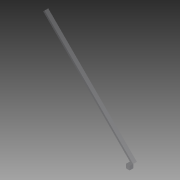
# Autodesk Inventor part: Mount
Saved by Autodesk Inventor 2013 (Build 170138000, 138)
## iProperties
Created: 2013-01-28
Part Number: Mount
Material: Polycarbonate, Clear
Document SubType Name: Modeling
Designer: Andrew Toennies
Density: 1.2 g/cm^3
Mass: 4.54796 g
Surface Area: 35.2548 cm^2
Volume: 3.78996 cm^3
Author: Andrew Toennies
Autodesk Inventor part; units mm, degrees
ref_plane "YZ Plane" through (0, 0, 0) normal (1, 0, 0) x (0, 1, 0)
ref_plane "XZ Plane" through (0, 0, 0) normal (0, 1, 0) x (-1, 0, 0)
ref_plane "XY Plane" through (0, 0, 0) normal (0, 0, 1) x (1, 0, 0)
sketch "Sketch1" plane through (0, 0, 0) normal (0, 0, 1) x (1, 0, 0)
  line L0 (-136.6846, 154.6451) -> (-138.9296, 152.4)
  line L1 (0, 0) -> (0, -6.35)
  line L2 (0, -6.35) -> (6.35, -6.35)
  line L3 (6.35, -6.35) -> (6.35, 0)
  line L4 (6.35, 0) -> (10.6475, 4.2975)
  line L5 (-108.1483, 123.0933) -> (17.5753, -2.6303) projected
  line L6 (10.6475, 4.2975) -> (-108.1483, 123.0933)
  line L7 (-108.1483, 123.0933) -> (-110.3933, 120.8483)
  line L8 (-110.3933, 120.8483) -> (5.2275, 5.2275)
  line L9 (0, 0) -> (5.2275, 5.2275)
  dimension "d2" = 3.175
  constraints: 18 end point, 3 perpendicular, 2 vertical, 1 horizontal, 1 point on line, 9 other
  measures "d2" distance of L5.start L7.end
extrude "Extrusion1" add sketch "Sketch1" along normal blind 6.35
body "Solid1"
